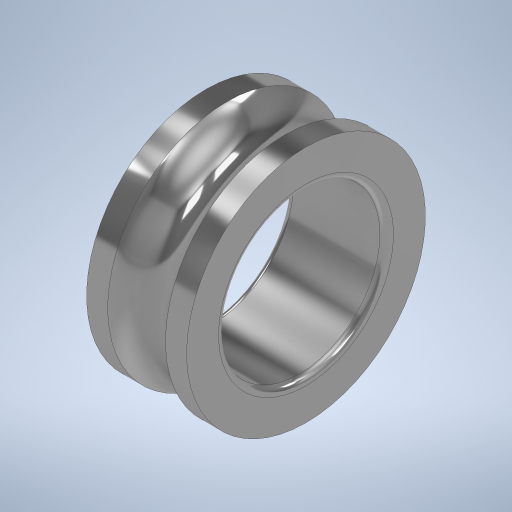
# Autodesk Inventor part: Inner Ring
Saved by Autodesk Inventor 2023 (Build 270158000, 158)
## iProperties
Created: 2023-03-23
Part Number: Inner Ring
Material: Generic
Document SubType Name: Modeling
Designer: CASPER
Density: 1 g/cm^3
Appearance: Chrome - Polished Black
Author: CASPER
Autodesk Inventor part; units mm, degrees
ref_plane "YZ Plane" through (0, 0, 0) normal (1, 0, 0) x (0, 1, 0)
ref_plane "XZ Plane" through (0, 0, 0) normal (0, 1, 0) x (-1, 0, 0)
ref_plane "XY Plane" through (0, 0, 0) normal (0, 0, 1) x (1, 0, 0)
sketch "Sketch1" plane through (0, 0, 0) normal (0, 0, 1) x (1, 0, 0)
  line L0 (-1.55, 3.7) -> (1.55, 3.7)
  line L1 (1.55, 3.7) -> (1.55, 2.5)
  line L2 (1.55, 2.5) -> (-1.55, 2.5)
  line L3 (-1.55, 2.5) -> (-1.55, 3.7)
  arc A0 (-0.8944, 3.7) -> (0.8944, 3.7) centre (0, 4.5) ccw
  line L4 (-2.17, 0) -> (2.17, 0) projected
  point P0 (0, 0)
  point P1 (0, 2.5)
  dimension "d0" = 3.1
  dimension "d1" = 1.2
  dimension "d2" = 1.55
  dimension "d3" = 2.5
  dimension "d4" = 0.8
  dimension "d5" = 1.2
  constraints: 8 end point, 2 parallel, 2 point on circle, 2 point on line, 1 centre point, 1 horizontal, 1 midpoint, 1 perpendicular, 1 vertical alignment
  measures "d0" distance of L0.start L0.end
  measures "d1" distance of L2.end L0.start
  measures "d2" horizontal distance of point (0, 0) L2.end
  measures "d3" distance of point (0, 0) point (0, 2.5)
  measures "d4" distance from line of L0 A0.centre
  measures "d5" radius of A0
revolve "Revolution1" add sketch "Sketch1" angle 360 about axis through (-10, 0, 0) along (1, 0, 0) contours L0 A0 L1 L2 L3
fillet "Fillet1" radius 0.21 2 edges at (1.55, -2.5, 0) (-1.55, -2.5, 0)
body "Solid1"
